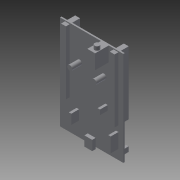
# Autodesk Inventor part: discovery
Saved by Autodesk Inventor 2014 SP1 (Build 180222100, 222)
## iProperties
Created: 2015-02-03
Part Number: discovery
Material: Générique
Document SubType Name: Modeling
Designer: astralien3000
Density: 1 g/cm^3
Appearance: Par défaut
Author: astralien3000
Autodesk Inventor part; units mm, degrees
ref_plane "YZ Plane" through (0, 0, 0) normal (1, 0, 0) x (0, 1, 0)
ref_plane "XZ Plane" through (0, 0, 0) normal (0, 1, 0) x (-1, 0, 0)
ref_plane "XY Plane" through (0, 0, 0) normal (0, 0, 1) x (1, 0, 0)
sketch "Esquisse1" plane through (0, 0, 0) normal (0, 1, 0) x (-1, 0, 0)
  line L0 (-32.5, 48.5) -> (32.5, 48.5)
  line L1 (32.5, 48.5) -> (32.5, -48.5)
  line L2 (32.5, -48.5) -> (-32.5, -48.5)
  line L3 (-32.5, -48.5) -> (-32.5, 48.5)
  point P0 (0, 0)
  dimension "d0" = 65
  dimension "d1" = 97
  dimension "d2" = 32.5
  dimension "d3" = 48.5
  constraints: 8 end point, 2 parallel, 1 horizontal, 1 perpendicular
  measures "d0" distance of L0.start L0.end
  measures "d1" distance of L0.end L1.end
  measures "d2" distance from line of L1 point (0, 0)
  measures "d3" distance from line of point (0, 0) L2
extrude "Extrusion1" add sketch "Esquisse1" along normal blind 1.5
sketch "Esquisse2" plane through (0, 1.5, 0) normal (0, 1, 0) x (1, 0, 0)
  line L0 (-32.5, -48.5) -> (32.5, -48.5) projected
  line L1 (32.5, -48.5) -> (32.5, 48.5) projected
  line L2 (-32.5, 48.5) -> (-32.5, -48.5) projected
  line L3 (-27.5, 17.5) -> (-22.5, 17.5)
  line L4 (-22.5, 17.5) -> (-22.5, -47.5)
  line L5 (-22.5, -47.5) -> (-27.5, -47.5)
  line L6 (-27.5, -47.5) -> (-27.5, 17.5)
  line L7 (22.5, 17.5) -> (27.5, 17.5)
  line L8 (27.5, 17.5) -> (27.5, -47.5)
  line L9 (27.5, -47.5) -> (22.5, -47.5)
  line L10 (22.5, -47.5) -> (22.5, 17.5)
  point P0 (0, 0)
  dimension "d6" = 5
  dimension "d7" = 5
  dimension "d8" = 65
  dimension "d9" = 5
  dimension "d10" = 5
  dimension "d11" = 1
  constraints: 16 end point, 4 parallel, 2 collinear, 2 horizontal, 2 perpendicular
  measures "d6" distance of L3.start L3.end
  measures "d7" distance of L7.start L7.end
  measures "d8" distance of L5.end L3.start
  measures "d9" distance between parallel lines of L2 L6
  measures "d10" distance between parallel lines of L1 L8
  measures "d11" distance between parallel lines of L0 L5
extrude "Extrusion2" add sketch "Esquisse2" along normal blind 9 and the other way blind 5.5
sketch "Esquisse3" plane through (0, 0, 0) normal (0, -1, 0) x (1, 0, 0)
  line L0 (32.5, 48.5) -> (-32.5, 48.5) projected
  line L1 (32.5, -48.5) -> (32.5, 48.5) projected
  line L2 (9.5, 48.5) -> (17.5, 48.5)
  line L3 (17.5, 48.5) -> (17.5, 33.5)
  line L4 (17.5, 33.5) -> (9.5, 33.5)
  line L5 (9.5, 33.5) -> (9.5, 48.5)
  point P0 (0, 0)
  dimension "d16" = 15
  dimension "d17" = 8
  dimension "d18" = 15
  constraints: 8 end point, 2 parallel, 1 horizontal, 1 perpendicular, 1 point on line
  measures "d16" distance of L4.end L2.start
  measures "d17" distance of L3.end L4.end
  measures "d18" distance between parallel lines of L1 L3
extrude "Extrusion3" add sketch "Esquisse3" along normal blind 14
sketch "Esquisse4" plane through (-32.5, 1.5, 48.5) normal (0, 0, 1) x (1, 0, 0)
  line L0 (50, -15.5) -> (42, -15.5) projected
  line L1 (50, -1.5) -> (50, -15.5) projected
  circle A0 centre (47, -10.5) radius 2.5
  point P0 (32.5, -1.5)
  dimension "d21" = 5
  dimension "d22" = 5
  dimension "d23" = 3
  constraints: 1 centre point
  measures "d21" distance from line of L0 A0.centre
  measures "d22" diameter of A0
  measures "d23" distance from line of L1 A0.centre
extrude "Extrusion4" add sketch "Esquisse4" along normal blind 4
sketch "Esquisse5" plane through (0, 0, 0) normal (0, -1, 0) x (1, 0, 0)
  line L0 (9.5, 48.5) -> (-32.5, 48.5) projected
  line L1 (-32.5, 48.5) -> (-32.5, -48.5) projected
  line L2 (32.5, -48.5) -> (32.5, 48.5) projected
  line L3 (32.5, 48.5) -> (17.5, 48.5) projected
  circle A0 centre (-12.5, 18.5) radius 2.5
  circle A1 centre (12.5, 18.5) radius 2.5
  point P0 (0, 0)
  dimension "d26" = 30
  dimension "d27" = 30
  dimension "d28" = 25
  dimension "d29" = 20
  dimension "d30" = 65
  dimension "d31" = 5
  dimension "d32" = 5
  constraints: 2 centre point
  measures "d26" distance from line of L0 A0.centre
  measures "d27" distance from line of L3 A1.centre
  measures "d28" distance of A1.centre A0.centre
  measures "d29" distance from line of L1 A0.centre
  measures "d30" distance between parallel lines of L2 L1
  measures "d31" diameter of A0
  measures "d32" diameter of A1
extrude "Extrusion5" add sketch "Esquisse5" along normal blind 10
sketch "Esquisse6" plane through (0, 0, 0) normal (0, -1, 0) x (1, 0, 0)
  line L0 (-32.5, 48.5) -> (-32.5, -48.5) projected
  line L1 (-32.5, -48.5) -> (32.5, -48.5) projected
  line L2 (32.5, -48.5) -> (32.5, 48.5) projected
  line L3 (27.5, -17.5) -> (22.5, -17.5) projected
  line L4 (22.5, -17.5) -> (22.5, 47.5) projected
  line L5 (25, -23.5) -> (27.5, -23.5)
  line L6 (27.5, -23.5) -> (27.5, -38.5)
  line L7 (27.5, -38.5) -> (25, -38.5)
  line L8 (25, -38.5) -> (25, -23.5)
  line L9 (-15.5, -23.5) -> (-13, -23.5)
  line L10 (-13, -23.5) -> (-13, -33.5)
  line L11 (-13, -33.5) -> (-15.5, -33.5)
  line L12 (-15.5, -33.5) -> (-15.5, -23.5)
  line L13 (14, -5) -> (16.5, -5)
  line L14 (16.5, -5) -> (16.5, -10)
  line L15 (16.5, -10) -> (14, -10)
  line L16 (14, -10) -> (14, -5)
  point P0 (0, 0)
  dimension "d35" = 2.5
  dimension "d36" = 2.5
  dimension "d37" = 2.5
  dimension "d38" = 10
  dimension "d39" = 5
  dimension "d40" = 15
  dimension "d41" = 5
  dimension "d42" = 17
  dimension "d43" = 6
  dimension "d44" = 10
  dimension "d45" = 15
  dimension "d46" = 7.5
  constraints: 24 end point, 6 parallel, 3 horizontal, 3 perpendicular
  measures "d35" distance of L5.start L5.end
  measures "d36" distance of L9.start L9.end
  measures "d37" distance of L13.start L13.end
  measures "d38" distance of L11.end L9.start
  measures "d39" distance of L13.end L14.end
  measures "d40" distance of L5.end L6.end
  measures "d41" distance between parallel lines of L2 L6
  measures "d42" distance between parallel lines of L0 L12
  measures "d43" distance between parallel lines of L4 L14
  measures "d44" distance between parallel lines of L1 L7
  measures "d45" distance between parallel lines of L1 L11
  measures "d46" distance between parallel lines of L3 L15
extrude "Extrusion6" add sketch "Esquisse6" along normal blind 8
sketch "Esquisse7" plane through (0, 0, 0) normal (0, -1, 0) x (1, 0, 0)
  line L0 (-32.5, 48.5) -> (-32.5, -48.5) projected
  line L1 (-32.5, -48.5) -> (32.5, -48.5) projected
  line L2 (-4, -40.5) -> (4, -40.5)
  line L3 (4, -40.5) -> (4, -50.5)
  line L4 (4, -50.5) -> (-4, -50.5)
  line L5 (-4, -50.5) -> (-4, -40.5)
  point P0 (0, 0)
  dimension "d49" = 10
  dimension "d50" = 8
  dimension "d51" = 65
  dimension "d52" = 28.5
  dimension "d53" = 2
  constraints: 8 end point, 2 parallel, 1 horizontal, 1 perpendicular
  measures "d49" distance of L4.end L2.start
  measures "d50" distance of L2.start L2.end
  measures "d51" distance of L0.end L1.end
  measures "d52" distance between parallel lines of L0 L5
  measures "d53" distance between parallel lines of L1 L4
extrude "Extrusion7" add sketch "Esquisse7" along normal blind 3.5
sketch "Esquisse8" plane through (0, 1.5, 0) normal (0, 1, 0) x (1, 0, 0)
  line L0 (32.5, -48.5) -> (32.5, 48.5) projected
  line L1 (32.5, 48.5) -> (-32.5, 48.5) projected
  line L2 (-32.5, 48.5) -> (-32.5, -48.5) projected
  line L3 (-27.5, 46.5) -> (-25, 46.5)
  line L4 (-25, 46.5) -> (-25, 41.5)
  line L5 (-25, 41.5) -> (-27.5, 41.5)
  line L6 (-27.5, 41.5) -> (-27.5, 46.5)
  line L7 (25, 46.5) -> (27.5, 46.5)
  line L8 (27.5, 46.5) -> (27.5, 41.5)
  line L9 (27.5, 41.5) -> (25, 41.5)
  line L10 (25, 41.5) -> (25, 46.5)
  point P0 (0, 0)
  dimension "d56" = 2.5
  dimension "d57" = 2.5
  dimension "d58" = 5
  dimension "d59" = 5
  dimension "d60" = 2
  dimension "d61" = 2
  dimension "d62" = 5
  dimension "d63" = 5
  constraints: 16 end point, 4 parallel, 2 horizontal, 2 perpendicular
  measures "d56" distance of L8.end L9.end
  measures "d57" distance of L4.end L5.end
  measures "d58" distance of L7.end L8.end
  measures "d59" distance of L5.end L3.start
  measures "d60" distance between parallel lines of L1 L7
  measures "d61" distance between parallel lines of L1 L3
  measures "d62" distance between parallel lines of L8 L0
  measures "d63" distance between parallel lines of L2 L6
extrude "Extrusion8" add sketch "Esquisse8" along normal blind 9
equation "\"d2\" = 0.5 * d0"
equation "\"d3\" = 0.5 * d1"
equation "\"d7\" = d6"
equation "\"d9\" = d6"
equation "\"d10\" = d9"
equation "\"d27\" = d26"
equation "\"d29\" = -0.5 * d28 + 0.5 * d30"
equation "\"d32\" = d31"
equation "\"d52\" = -0.5 * d50 + 0.5 * d51"
equation "\"d57\" = d56"
equation "\"d61\" = d60"
equation "\"d63\" = d62"
